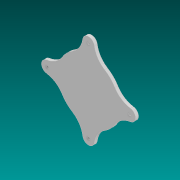
# Autodesk Inventor part: onderkant base
Saved by Autodesk Inventor 2020.2 (Build 242310000, 310)
## iProperties
Created: 2020-05-18
Part Number: onderkant base
Material: Generic
Document SubType Name: Modeling
Designer: Svend
Density: 1 g/cm^3
Appearance: Default
Author: Svend
Autodesk Inventor part; units mm, degrees
ref_plane "YZ Plane" through (0, 0, 0) normal (1, 0, 0) x (0, 1, 0)
ref_plane "XZ Plane" through (0, 0, 0) normal (0, 1, 0) x (-1, 0, 0)
ref_plane "XY Plane" through (0, 0, 0) normal (0, 0, 1) x (1, 0, 0)
sketch "Sketch1" plane through (0, 0, 0) normal (0, 0, 1) x (1, 0, 0)
  circle A0 centre (0, 0) radius 105
  circle A1 centre (140, 0) radius 4
  circle A2 centre (140, 0) radius 20
  arc A3 (89.5312, 54.8558) -> (142.8383, 19.7976) centre (153.4821, 94.0385) ccw
  arc A4 (142.8383, -19.7976) -> (89.5312, -54.8558) centre (153.4821, -94.0385) ccw
  circle A5 centre (0, 140) radius 4
  circle A6 centre (0, 140) radius 20
  arc A7 (19.7976, 142.8383) -> (54.8558, 89.5312) centre (94.0385, 153.4821) ccw
  arc A8 (-54.8558, 89.5312) -> (-19.7976, 142.8383) centre (-94.0385, 153.4821) ccw
  circle A9 centre (-140, 0) radius 4
  circle A10 centre (-140, 0) radius 20
  arc A11 (-142.8383, 19.7976) -> (-89.5312, 54.8558) centre (-153.4821, 94.0385) ccw
  arc A12 (-89.5312, -54.8558) -> (-142.8383, -19.7976) centre (-153.4821, -94.0385) ccw
  circle A13 centre (0, -140) radius 4
  circle A14 centre (0, -140) radius 20
  arc A15 (-19.7976, -142.8383) -> (-54.8558, -89.5312) centre (-94.0385, -153.4821) ccw
  arc A16 (54.8558, -89.5313) -> (19.7976, -142.8383) centre (94.0385, -153.4821) ccw
  point P0 (-54.8558, 89.5312)
  point P1 (-89.5312, 54.8558)
  point P2 (-54.8558, -89.5312)
  point P3 (54.8558, -89.5312)
  dimension "d0" = 210
  dimension "d1" = 8
  dimension "d2" = 40
  dimension "d3" = 140
  dimension "d4" = 75
  dimension "d7" = 360
  constraints: 26 point on circle, 17 centre point, 5 coincident, 4 tangent, 1 equal radius, 1 horizontal alignment, 49 other
  measures "d0" diameter of A0
  measures "d1" diameter of A1
  measures "d2" diameter of A2
  measures "d3" distance of point (0, 0) A1.centre
  measures "d4" radius of A3
extrude "Extrusion1" add sketch "Sketch1" along normal blind 10
sketch "Sketch2" plane through (0, 0, 0) normal (1, 0, 0) x (0, 1, 0)
  line L0 (-89.5312, 10) -> (-142.8383, 10) projected
  line L1 (-142.8383, 10) -> (-142.8383, 10) projected
  line L2 (-142.8383, 10) -> (-89.5312, 10) projected
  line L3 (-89.5312, 10) -> (-54.8558, 10) projected
  line L4 (-54.8558, 10) -> (-19.7976, 10) projected
  line L5 (-19.7976, 10) -> (19.7976, 10) projected
  line L6 (19.7976, 10) -> (54.8558, 10) projected
  line L7 (54.8558, 10) -> (89.5312, 10) projected
  line L8 (89.5312, 10) -> (142.8383, 10) projected
  line L9 (142.8383, 10) -> (142.8383, 10) projected
  line L10 (142.8383, 10) -> (89.5312, 10) projected
  line L11 (89.5312, 10) -> (54.8558, 10) projected
  line L12 (54.8558, 10) -> (19.7976, 10) projected
  line L13 (19.7976, 10) -> (-19.7976, 10) projected
  line L14 (-19.7976, 10) -> (-54.8558, 10) projected
  line L15 (-54.8558, 10) -> (-89.5312, 10) projected
  line L16 (-4, 10) -> (4, 10) projected
  line L17 (136, 10) -> (144, 10) projected
  line L18 (-4, 10) -> (4, 10) projected
  line L19 (-144, 10) -> (-136, 10) projected
  line L20 (-89.5312, 0) -> (-142.8383, 0) projected
  line L21 (-54.8558, 0) -> (-89.5312, 0) projected
  line L22 (-19.7976, 0) -> (-54.8558, 0) projected
  line L23 (19.7976, 0) -> (-19.7976, 0) projected
  line L24 (54.8558, 0) -> (19.7976, 0) projected
  line L25 (89.5312, 0) -> (54.8558, 0) projected
  line L26 (142.8383, 0) -> (89.5312, 0) projected
  line L27 (142.8383, 0) -> (142.8383, 0) projected
  line L28 (89.5312, 0) -> (142.8383, 0) projected
  line L29 (54.8558, 0) -> (89.5312, 0) projected
  line L30 (19.7976, 0) -> (54.8558, 0) projected
  line L31 (-19.7976, 0) -> (19.7976, 0) projected
  line L32 (-54.8558, 0) -> (-19.7976, 0) projected
  line L33 (-89.5312, 0) -> (-54.8558, 0) projected
  line L34 (-142.8383, 0) -> (-89.5312, 0) projected
  line L35 (-142.8383, 0) -> (-142.8383, 0) projected
  line L36 (-4, 0) -> (4, 0) projected
  line L37 (136, 0) -> (144, 0) projected
  line L38 (-4, 0) -> (4, 0) projected
  line L39 (-144, 0) -> (-136, 0) projected
  circle A0 centre (-95, -1) radius 7.5
  line L40 (0, 0) -> (0, 10)
  dimension "d11" = 15
  dimension "d12" = 1
  dimension "d13" = 95
  constraints: 2 end point, 1 centre point, 1 midpoint
  measures "d11" diameter of A0
  measures "d12" distance from line of L20 A0.centre
  measures "d13" horizontal distance of L40.start A0.centre
revolve "Revolution1" cut sketch "Sketch2" angle 360 about axis through (0, 0, 0) along (0, 0, 1)
body "Solid1"
